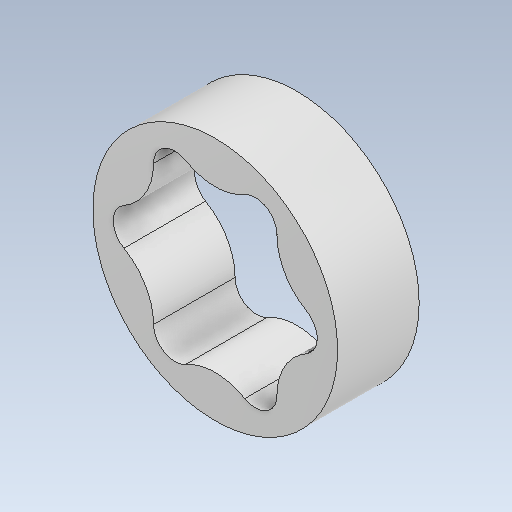
# Autodesk Inventor part: 3ギア接続部外
Saved by Autodesk Inventor 2020.4 (Build 244396000, 396)
## iProperties
Created: 2021-05-01
Part Number: 3ギア接続部外
Material: アルミニウム 2014-T4
Document SubType Name: Modeling
Designer: happy
Density: 2.8 g/cm^3
Appearance: サテン
Mass: 0.577001 g
Surface Area: 3.79496 cm^2
Volume: 0.206072 cm^3
Author: happy
Autodesk Inventor part; units mm, degrees
ref_plane "YZ Plane" through (0, 0, 0) normal (1, 0, 0) x (0, 1, 0)
ref_plane "XZ Plane" through (0, 0, 0) normal (0, 1, 0) x (-1, 0, 0)
ref_plane "XY Plane" through (0, 0, 0) normal (0, 0, 1) x (1, 0, 0)
sketch "スケッチ1" plane through (0, 0, 0) normal (0, 0, 1) x (1, 0, 0)
  circle A0 centre (148.5, 105.0001) radius 5 construction
  line L0 (146, 109.3303) -> (151, 109.3303) construction
  line L1 (151, 109.3303) -> (153.5, 105.0001) construction
  line L2 (153.5, 105.0001) -> (151, 100.67) construction
  line L3 (151, 100.67) -> (146, 100.67) construction
  line L4 (146, 100.67) -> (143.5, 105.0001) construction
  line L5 (143.5, 105.0001) -> (146, 109.3303) construction
  arc A1 (147.05, 109.3303) -> (145.475, 108.4209) centre (146.525, 108.4209) ccw
  arc A2 (144.025, 105.9095) -> (144.025, 104.0908) centre (144.55, 105.0001) ccw
  arc A3 (145.475, 101.5793) -> (147.05, 100.67) centre (146.525, 101.5793) ccw
  arc A4 (149.95, 100.67) -> (151.525, 101.5793) centre (150.475, 101.5793) ccw
  arc A5 (152.975, 104.0908) -> (152.975, 105.9095) centre (152.45, 105.0001) ccw
  arc A6 (151.525, 108.4209) -> (149.95, 109.3303) centre (150.475, 108.4209) ccw
  arc A7 (147.05, 109.3303) -> (149.95, 109.3303) centre (148.5, 111.8417) ccw
  arc A8 (144.025, 105.9095) -> (145.475, 108.4209) centre (142.575, 108.4209) ccw
  arc A9 (145.475, 101.5793) -> (144.025, 104.0908) centre (142.575, 101.5793) ccw
  arc A10 (149.95, 100.67) -> (147.05, 100.67) centre (148.5, 98.1585) ccw
  arc A11 (152.975, 104.0908) -> (151.525, 101.5793) centre (154.425, 101.5793) ccw
  arc A12 (151.525, 108.4209) -> (152.975, 105.9095) centre (154.425, 108.4209) ccw
  circle A13 centre (148.5, 105.0001) radius 2 construction
  circle A14 centre (148.5, 105.0001) radius 6
  point P0 (0, 0)
  point P1 (146, 100.67)
  point P2 (151, 100.67)
  point P3 (153.5, 105.0001)
  point P4 (145.475, 101.5793)
  point P5 (144.025, 104.0908)
  point P6 (144.025, 105.9095)
  point P7 (145.475, 108.4209)
  point P8 (151.525, 108.4209)
  point P9 (152.975, 105.9095)
  point P10 (152.975, 104.0908)
  point P11 (151.525, 101.5793)
  point P12 (147.05, 100.67)
  dimension "d4" = 10
  dimension "d5" = 360
  dimension "d6" = 360
  dimension "d7" = 1.05
  dimension "d8" = 4
  dimension "d9" = 12
  constraints: 30 point on circle, 14 centre point, 12 end point, 4 coincident, 2 point on line, 2 tangent, 1 horizontal alignment, 73 other
  measures "d7" radius of A1
  measures "d8" diameter of A13
  measures "d9" diameter of A14
extrude "押し出し1" add sketch "スケッチ1" along normal blind 4
